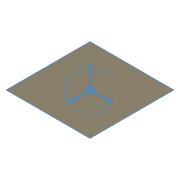
# Autodesk Inventor part: Floor
Saved by Autodesk Inventor 2012 (Build 160160000, 160)
## iProperties
Created: 2012-01-09
Part Number: Floor
Material: Wood (Birch)
Document SubType Name: Modeling
Designer: JesseK
Density: 0.00191488 g/cm^3
Mass: 4.53592 g
Surface Area: 186549 cm^2
Volume: 2368.78 cm^3
Author: JesseK
Autodesk Inventor part; units mm, degrees
ref_plane "YZ Plane" through (0, 0, 0) normal (1, 0, 0) x (0, 1, 0)
ref_plane "XZ Plane" through (0, 0, 0) normal (0, 1, 0) x (-1, 0, 0)
ref_plane "XY Plane" through (0, 0, 0) normal (0, 0, 1) x (1, 0, 0)
sketch "Sketch1" plane through (0, 0, 0) normal (0, 0, 1) x (1, 0, 0)
  line L0 (0, 0) -> (3048, 0)
  line L1 (3048, 0) -> (3048, 3.175)
  line L2 (3048, 3.175) -> (0, 3.175)
  line L3 (0, 3.175) -> (0, 0)
  dimension "d0" = 3048
  dimension "d1" = 3.175
  constraints: 8 end point, 2 parallel, 1 horizontal, 1 perpendicular
  measures "d0" distance of L1.end L2.end
  measures "d1" distance of L2.end L0.start
extrude "Extrusion1" add sketch "Sketch1" along normal blind 3048
shell "Shell1" thickness 0.254 removed faces 1 at (1016, 0, 2032)
body "Solid1"
